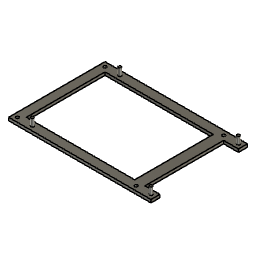
PCB_Holder_ShiftLeft v2 (Autodesk Fusion 360 design; units mm, degrees)
Autodesk Fusion 360 part; units mm, degrees
note: some values were not read from the file. Chosen so that the rebuilt part matches the saved one: which face or edge a step refers to; which pieces of a blend or face edit are solid.
sketch "Sketch1" plane through (0, 0, 0) normal (0, 0, 1) x (1, 0, 0)
  line L0 (0, 180) -> (180, 180)
  line L1 (180, 180) -> (180, 0)
  line L2 (180, 0) -> (0, 0)
  line L3 (0, 0) -> (0, 180)
  line L4 (10, 170) -> (170, 170)
  line L5 (170, 170) -> (170, 10)
  line L6 (170, 10) -> (10, 10)
  line L7 (10, 10) -> (10, 170)
  constraint horizontal L0
  constraint vertical L1
  constraint horizontal L2
  constraint vertical L3
  constraint horizontal L4
  constraint vertical L5
  constraint horizontal L6
  constraint vertical L7
sketch "Sketch2" plane through (0, 0, 4) normal (0, 0, 1) x (-1, 0, 0)
  line L0 (-170, -10) -> (-10, -10)
  line L1 (-10, -10) -> (-10, -170)
  line L2 (-10, -170) -> (-170, -170)
  line L3 (-170, -170) -> (-170, -10)
  line L4 (0, 0) -> (-180, 0)
  line L5 (-180, 0) -> (-180, -180)
  line L6 (-180, -180) -> (0, -180)
  line L7 (0, -180) -> (0, 0)
  circle A0 centre (-5, -5) radius 2
sketch "Sketch3" plane through (0, 0, 0) normal (0, 0, 1) x (1, 0, 0)
  line L0 (0, 0) -> (172, 0)
  line L1 (172, 0) -> (172, 130)
  line L2 (172, 130) -> (0, 130)
  line L3 (0, 130) -> (0, 0)
  line L4 (12, 12) -> (158, 12)
  line L5 (158, 12) -> (158, 118)
  line L6 (158, 118) -> (12, 118)
  line L7 (12, 118) -> (12, 12)
  dimension "d5" = 172
  dimension "d6" = 130
  constraint horizontal L0
  constraint vertical L1
  constraint horizontal L2
  constraint vertical L3
  constraint coincident L0.start L3.end
  constraint horizontal L4
  constraint vertical L5
  constraint horizontal L6
  constraint vertical L7
  measures "d5" distance of L0.start L0.end
  measures "d6" distance of L0.start L2.end
extrude "Extrude3" add sketch "Sketch3" along normal blind 4
sketch "Sketch4" plane through (0, 0, 4) normal (0, 0, 1) x (-1, 0, 0)
  line L0 (-12, -12) -> (-12, -118)
  line L1 (-12, -118) -> (-158, -118)
  line L2 (-158, -118) -> (-158, -12)
  line L3 (-158, -12) -> (-12, -12)
  line L4 (0, -130) -> (0, 0)
  line L5 (0, 0) -> (-172, 0)
  line L6 (-172, 0) -> (-172, -130)
  line L7 (-172, -130) -> (0, -130)
  circle A0 centre (-6, -6) radius 4
extrude "Extrude4" add sketch "Sketch4" along normal blind 10 contours A0
sketch "Sketch5" plane through (0, 0, 4) normal (0, 0, 1) x (-1, 0, 0)
  circle A0 centre (-6, -6) radius 4
  line L0 (-12, -12) -> (-12, -118)
  line L1 (-12, -118) -> (-158, -118)
  line L2 (-158, -118) -> (-158, -12)
  line L3 (-158, -12) -> (-12, -12)
  line L4 (0, -130) -> (0, 0)
  line L5 (0, 0) -> (-172, 0)
  line L6 (-172, 0) -> (-172, -130)
  line L7 (-172, -130) -> (0, -130)
  circle A1 centre (-6, -124) radius 4
extrude "Extrude5" add sketch "Sketch5" along normal blind 10 contours A1
sketch "Sketch6" plane through (0, 0, 0) normal (0, 0, 1) x (1, 0, 0)
sketch "Sketch7" plane through (0, 0, 4) normal (0, 0, 1) x (-1, 0, 0)
  circle A0 centre (-6, -124) radius 4
  circle A1 centre (-6, -6) radius 4
  line L0 (-12, -12) -> (-12, -118)
  line L1 (-12, -118) -> (-158, -118)
  line L2 (-158, -118) -> (-158, -12)
  line L3 (-158, -12) -> (-12, -12)
  line L4 (0, -130) -> (0, 0)
  line L5 (0, 0) -> (-172, 0)
  line L6 (-172, 0) -> (-172, -130)
  line L7 (-172, -130) -> (0, -130)
  circle A2 centre (-166, -124) radius 4
extrude "Extrude6" add sketch "Sketch7" along normal blind 10 contours A2
sketch "Sketch8" plane through (0, 0, 4) normal (0, 0, 1) x (-1, 0, 0)
  circle A0 centre (-166, -124) radius 4
  circle A1 centre (-6, -124) radius 4
  circle A2 centre (-6, -6) radius 4
  line L0 (-12, -12) -> (-12, -118)
  line L1 (-12, -118) -> (-158, -118)
  line L2 (-158, -118) -> (-158, -12)
  line L3 (-158, -12) -> (-12, -12)
  line L4 (0, -130) -> (0, 0)
  line L5 (0, 0) -> (-172, 0)
  line L6 (-172, 0) -> (-172, -130)
  line L7 (-172, -130) -> (0, -130)
  circle A3 centre (-166, -6) radius 4
extrude "Extrude7" add sketch "Sketch8" along normal blind 10 contours A3
sketch "Sketch9" plane through (0, 0, 0) normal (0, 0, 1) x (1, 0, 0)
  line L0 (0, 0) -> (10, 0)
  line L1 (10, 0) -> (10, -26)
  line L2 (10, -26) -> (0, -26)
  line L3 (0, -26) -> (0, 0)
  constraint horizontal L0
  constraint vertical L1
  constraint horizontal L2
  constraint vertical L3
  constraint coincident L0.start L3.end
extrude "Extrude8" add sketch "Sketch9" along normal blind 4
sketch "Sketch10" plane through (0, 0, 0) normal (0, 0, 1) x (1, 0, 0)
  line L0 (172, 0) -> (160, 0)
  line L1 (160, 0) -> (160, -26)
  line L2 (160, -26) -> (172, -26)
  line L3 (172, -26) -> (172, 0)
  constraint horizontal L0
  constraint vertical L1
  constraint horizontal L2
  constraint vertical L3
extrude "Extrude9" add sketch "Sketch10" along normal blind 4
sketch "Sketch11" plane through (0, 0, 0) normal (0, 0, 1) x (1, 0, 0)
  line L0 (0, 130) -> (12, 130)
  line L1 (12, 130) -> (12, 156)
  line L2 (12, 156) -> (0, 156)
  line L3 (0, 156) -> (0, 130)
  line L4 (172, 130) -> (160, 130)
  line L5 (160, 130) -> (160, 156)
  line L6 (160, 156) -> (172, 156)
  line L7 (172, 156) -> (172, 130)
  constraint horizontal L0
  constraint vertical L1
  constraint horizontal L2
  constraint vertical L3
  constraint horizontal L4
  constraint vertical L5
  constraint horizontal L6
  constraint vertical L7
extrude "Extrude10" add sketch "Sketch11" along normal blind 4
sketch "Sketch12" plane through (0, 0, 0) normal (0, 0, 1) x (1, 0, 0)
  line L0 (0, -26, 4) -> (-5, -26, 4)
  line L1 (-5, -26, 4) -> (-5, -14, 4)
  line L2 (-5, -14, 4) -> (0, -14, 4)
  line L3 (0, -14, 4) -> (0, -26, 4)
  line L4 (172, -26, 4) -> (177, -26, 4)
  line L5 (177, -26, 4) -> (177, -14, 4)
  line L6 (177, -14, 4) -> (172, -14, 4)
  line L7 (172, -14, 4) -> (172, -26, 4)
  line L8 (172, 156, 4) -> (177, 156, 4)
  line L9 (177, 156, 4) -> (177, 144, 4)
  line L10 (177, 144, 4) -> (172, 144, 4)
  line L11 (172, 144, 4) -> (172, 156, 4)
  line L12 (0, 156, 4) -> (-5, 156, 4)
  line L13 (-5, 156, 4) -> (-5, 144, 4)
  line L14 (-5, 144, 4) -> (0, 144, 4)
  line L15 (0, 144, 4) -> (0, 156, 4)
sketch "Sketch12 (curves 4 mm off its plane)" plane through (0, 0, 4) normal (0, 0, 1) x (1, 0, 0)
  line L0 (0, -26) -> (-5, -26)
  line L1 (-5, -26) -> (-5, -14)
  line L2 (-5, -14) -> (0, -14)
  line L3 (0, -14) -> (0, -26)
  line L4 (172, -26) -> (177, -26)
  line L5 (177, -26) -> (177, -14)
  line L6 (177, -14) -> (172, -14)
  line L7 (172, -14) -> (172, -26)
  line L8 (172, 156) -> (177, 156)
  line L9 (177, 156) -> (177, 144)
  line L10 (177, 144) -> (172, 144)
  line L11 (172, 144) -> (172, 156)
  line L12 (0, 156) -> (-5, 156)
  line L13 (-5, 156) -> (-5, 144)
  line L14 (-5, 144) -> (0, 144)
  line L15 (0, 144) -> (0, 156)
extrude "Extrude11" add sketch "Sketch12 (curves 4 mm off its plane)" against normal blind 4
sketch "Sketch13" plane through (0, 0, 0) normal (0, 0, -1) x (1, 0, 0)
  line L0 (12, -118) -> (12, -12)
  line L1 (12, -12) -> (158, -12)
  line L2 (158, -12) -> (158, -118)
  line L3 (158, -118) -> (12, -118)
  line L4 (-5, -156) -> (12, -156)
  line L5 (12, -156) -> (12, -130)
  line L6 (12, -130) -> (160, -130)
  line L7 (160, -130) -> (160, -156)
  line L8 (160, -156) -> (177, -156)
  line L9 (177, -156) -> (177, -144)
  line L10 (177, -144) -> (172, -144)
  line L11 (172, -144) -> (172, -130)
  line L12 (172, -130) -> (172, 0)
  line L13 (172, 0) -> (172, 14)
  line L14 (172, 14) -> (177, 14)
  line L15 (177, 14) -> (177, 26)
  line L16 (177, 26) -> (160, 26)
  line L17 (160, 26) -> (160, 0)
  line L18 (160, 0) -> (10, 0)
  line L19 (10, 0) -> (10, 26)
  line L20 (10, 26) -> (-5, 26)
  line L21 (-5, 26) -> (-5, 14)
  line L22 (-5, 14) -> (0, 14)
  line L23 (0, 14) -> (0, -144)
  line L24 (0, -144) -> (-5, -144)
  line L25 (-5, -144) -> (-5, -156)
  circle A0 centre (1, 20) radius 2
  circle A1 centre (171, 20) radius 2
extrude "Extrude12" cut sketch "Sketch13" against normal blind 4 contours A0 | A1
sketch "Sketch14" plane through (0, 0, 4) normal (0, 0, 1) x (-1, 0, 0)
  circle A0 centre (-1, 20) radius 2
  circle A1 centre (-171, 20) radius 2
  circle A2 centre (-166, -6) radius 4
  circle A3 centre (-166, -124) radius 4
  circle A4 centre (-6, -124) radius 4
  circle A5 centre (-6, -6) radius 4
  line L0 (-12, -12) -> (-12, -118)
  line L1 (-12, -118) -> (-158, -118)
  line L2 (-158, -118) -> (-158, -12)
  line L3 (-158, -12) -> (-12, -12)
  line L4 (0, -144) -> (0, 14)
  line L5 (0, 14) -> (5, 14)
  line L6 (5, 14) -> (5, 26)
  line L7 (5, 26) -> (-10, 26)
  line L8 (-10, 26) -> (-10, 0)
  line L9 (-10, 0) -> (-160, 0)
  line L10 (-160, 0) -> (-160, 26)
  line L11 (-160, 26) -> (-177, 26)
  line L12 (-177, 26) -> (-177, 14)
  line L13 (-177, 14) -> (-172, 14)
  line L14 (-172, 14) -> (-172, 0)
  line L15 (-172, 0) -> (-172, -130)
  line L16 (-172, -130) -> (-172, -144)
  line L17 (-172, -144) -> (-177, -144)
  line L18 (-177, -144) -> (-177, -156)
  line L19 (-177, -156) -> (-160, -156)
  line L20 (-160, -156) -> (-160, -130)
  line L21 (-160, -130) -> (-12, -130)
  line L22 (-12, -130) -> (-12, -156)
  line L23 (-12, -156) -> (5, -156)
  line L24 (5, -156) -> (5, -144)
  line L25 (5, -144) -> (0, -144)
  circle A6 centre (-1, -150) radius 2
  circle A7 centre (-171, -150) radius 2
extrude "Extrude13" cut sketch "Sketch14" against normal blind 4 contours A6 | A7
extrude "Extrude14" add 4 faces at (166.0996, 8.1156, 14) (167.2013, 123.4215, 14) (6.6074, 6.7617, 14) (7.1017, 125.1485, 14) along direction (0, 0, 1) blind 40
sketch "Sketch15" plane through (0, 0, 54) normal (0, 0, 1) x (-1, 0, 0)
  circle A0 centre (-166, -6) radius 4
  circle A1 centre (-166, -6) radius 2
  circle A2 centre (-166, -124) radius 2
  circle A3 centre (-6, -124) radius 2
  circle A4 centre (-6, -6) radius 2
  constraint concentric A0 A1
extrude "Extrude15" cut sketch "Sketch15" against normal blind 14 contours A1 | A2 | A3 | A4
extrude "Extrude16" add 1 faces at (4.9621, 123.6245, 40) along direction (0, 0, 1) blind 20
extrude "Extrude17" cut 1 faces at (4.9621, 123.6245, 60) along direction (0, 0, -1) blind 83
extrude "Extrude18" cut 1 faces at (6.5872, 5.8898, 40) along direction (0, 0, -1) blind 258
extrude "Extrude19" cut 1 faces at (166.2436, 6.8193, 40) along direction (0, 0, -1) blind 100
extrude "Extrude20" cut 1 faces at (166.9758, 124.4535, 40) along direction (0, 0, -1) blind 1000
delete_face "DeleteFace1" 1 faces at (2.0199, 6.3983, 20.6667)
delete_face "DeleteFace2" 1 faces at (8.7929, 126.8635, 37.3333)
delete_face "DeleteFace3" 1 faces at (165.3054, 120.0608, 20.6667)
delete_face "DeleteFace4" 1 faces at (165.5026, 9.969, 37.3333)
extrude "Extrude21" cut 1 faces at (165.6667, 156, 2.6667) along direction (0, -1, 0) blind 26
extrude "Extrude22" cut 1 faces at (6.3333, 156, 2.6667) along direction (0, -1, 0) blind 26
extrude "Extrude23" cut 1 faces at (165.6667, -26, 2.6667) along direction (0, 1, 0) blind 26
extrude "Extrude24" cut 1 faces at (5, -26, 1.3333) along direction (0, 1, 0) blind 26
sketch "Sketch16" plane through (0, 0, 0) normal (0, 0, 1) x (1, 0, 0)
  line L0 (172, 0) -> (206, 0)
  line L1 (206, 0) -> (206, 11.7)
  line L2 (206, 11.7) -> (172, 11.7)
  line L3 (172, 11.7) -> (172, 0)
  line L4 (172, 130) -> (206, 130)
  line L5 (206, 130) -> (206, 118)
  line L6 (206, 118) -> (172, 118)
  line L7 (172, 118) -> (172, 130)
  dimension "d54" = 34
  dimension "d55" = 34
  dimension "d56" = 12
  constraint horizontal L0
  constraint vertical L1
  constraint horizontal L2
  constraint vertical L3
  constraint horizontal L4
  constraint vertical L5
  constraint horizontal L6
  constraint vertical L7
  measures "d54" distance of L0.start L0.end
  measures "d55" distance of L4.start L4.end
  measures "d56" distance of L4.start L6.end
extrude "Extrude25" add sketch "Sketch16" along normal blind 4
sketch "Sketch17" plane through (0, 0, 0) normal (0, 0, 1) x (1, 0, 0)
extrude "Extrude26" add 1 faces at (194.6667, 11.7, 1.3333) along direction (0, 1, 0) blind 0.3
sketch "Sketch18" plane through (0, 0, 4) normal (0, 0, 1) x (-1, 0, 0)
  line L0 (0, 0) -> (-172, 0)
  line L1 (-172, 0) -> (-206, 0)
  line L2 (-206, 0) -> (-206, -12)
  line L3 (-206, -12) -> (-172, -12)
  line L4 (-172, -12) -> (-172, -118)
  line L5 (-172, -118) -> (-206, -118)
  line L6 (-206, -118) -> (-206, -130)
  line L7 (-206, -130) -> (-172, -130)
  line L8 (-172, -130) -> (0, -130)
  line L9 (0, -130) -> (0, 0)
  line L10 (-12, -12) -> (-12, -118)
  line L11 (-12, -118) -> (-158, -118)
  line L12 (-158, -118) -> (-158, -12)
  line L13 (-158, -12) -> (-12, -12)
  circle A0 centre (-6, -6) radius 2
  circle A1 centre (-6, -124) radius 2
  circle A2 centre (-166, -124) radius 2
  circle A3 centre (-166, -6) radius 2
  circle A4 centre (-200.0145, -6) radius 2
  circle A5 centre (-200, -124) radius 2
  dimension "d61" = 4
  dimension "d62" = 4
  measures "d61" diameter of A4
  measures "d62" diameter of A5
extrude "Extrude27" add sketch "Sketch18" along normal blind 10 contours A4 | A5
move_face "MoveFace1" to x (1, 0, 0) y (0, 1, 0) z (0, 0, 1) at (-0.15, 0, 0) 1 faces at (201.411, 4.5683, 10.6667)
move_face "MoveFace2" to x (1, 0, 0) y (0, 1, 0) z (0, 0, 1) at (0.135, 0, 0) 1 faces at (201.1879, 4.5004, 10.6667)
sketch "Sketch19" plane through (0, 0, 4) normal (0, 0, 1) x (-1, 0, 0)
  circle A0 centre (-200, -124) radius 2
  circle A1 centre (-199.9995, -6) radius 2
  line L0 (0, 0) -> (-172, 0)
  line L1 (-172, 0) -> (-206, 0)
  line L2 (-206, 0) -> (-206, -12)
  line L3 (-206, -12) -> (-172, -12)
  line L4 (-172, -12) -> (-172, -118)
  line L5 (-172, -118) -> (-206, -118)
  line L6 (-206, -118) -> (-206, -130)
  line L7 (-206, -130) -> (-172, -130)
  line L8 (-172, -130) -> (0, -130)
  line L9 (0, -130) -> (0, 0)
  line L10 (-12, -12) -> (-12, -118)
  line L11 (-12, -118) -> (-158, -118)
  line L12 (-158, -118) -> (-158, -12)
  line L13 (-158, -12) -> (-12, -12)
  circle A2 centre (-6, -6) radius 2
  circle A3 centre (-6, -124) radius 2
  circle A4 centre (-166, -124) radius 2
  circle A5 centre (-166, -6) radius 2
  circle A6 centre (-8, -6) radius 30
  circle A7 centre (-40, -6) radius 2
  circle A8 centre (-40, -124) radius 2
  dimension "d65" = 60
  constraint coincident A2 A6.centre
  measures "d65" diameter of A6
extrude "Extrude28" add sketch "Sketch19" along normal blind 10 contours A7 | A8
move_face "MoveFace3" to x (1, 0, 0) y (0, 1, 0) z (0, 0, 1) at (-20, 0, 0) 8 faces at (198.9149, 122.32, 10.6667) (38.0025, 124.0997, 10.6667) (201.3229, 4.5004, 10.6667) (39.4583, 4.0748, 10.6667) (199.363, 125.1034, 14) (41.0379, 123.6245, 14) (200.1569, 4.8074, 14) (39.5843, 6.3857, 14)
move_face "OffsetFaces1" offset -14 2 faces at (206, 126, 1.3333) (206, 8, 2.6667)
move_face "MoveFace4" to x (1, 0, 0) y (0, 1, 0) z (0, 0, 1) at (6, 0, 0) 8 faces at (178.8325, 122.3761, 7.3333) (18.0099, 123.8009, 10.6667) (181.3229, 4.5004, 10.6667) (18.0099, 5.8009, 10.6667) (180.6006, 124.2893, 14) (21.0379, 124.3755, 14) (179.3625, 5.8035, 14) (19.6465, 6.4433, 14)
